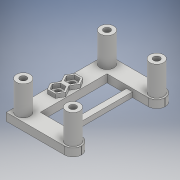
# Autodesk Inventor part: mountMount
Saved by Autodesk Inventor 2018 (Build 220112000, 112)
## iProperties
Created: 2018-05-09
Part Number: mountMount
Material: Generic
Document SubType Name: Modeling
Designer: s4321966
Density: 1 g/cm^3
Appearance: Default
Mass: 5.25986 g
Surface Area: 52.6128 cm^2
Volume: 5.25986 cm^3
Author: s4321966
Autodesk Inventor part; units mm, degrees
ref_plane "YZ Plane" through (0, 0, 0) normal (1, 0, 0) x (0, 1, 0)
ref_plane "XZ Plane" through (0, 0, 0) normal (0, 1, 0) x (-1, 0, 0)
ref_plane "XY Plane" through (0, 0, 0) normal (0, 0, 1) x (1, 0, 0)
sketch "Sketch1" plane through (0, 0, 0) normal (0, 0, 1) x (1, 0, 0)
  line L0 (0, 0) -> (41.5, 0)
  line L1 (41.5, 0) -> (41.5, -73)
  line L2 (41.5, -73) -> (0, -73)
  line L3 (0, -73) -> (0, 0)
  line L4 (0, -73) -> (3.11, -73)
  line L5 (0, -73) -> (3.11, -73) construction
  line L6 (3.11, -73) -> (3.11, -69.85)
  line L7 (3.11, -73) -> (6.26, -73) construction
  line L8 (3.11, -69.85) -> (14.54, -69.85)
  line L9 (14.54, -69.85) -> (19.65, -69.85)
  line L10 (19.65, -69.85) -> (31.08, -69.85)
  circle A0 centre (3.11, -69.85) radius 1.6
  circle A1 centre (14.54, -69.85) radius 1.6
  circle A2 centre (19.65, -69.85) radius 1.6
  circle A3 centre (31.08, -69.85) radius 1.6
  line L11 (3.11, -69.85) -> (3.11, -55.42)
  line L12 (3.11, -69.85) -> (17.54, -69.85) construction
  line L13 (0, -73) -> (4.33, -73)
  line L14 (0, -73) -> (4.33, -73) construction
  line L15 (4.33, -73) -> (4.33, -53.49)
  line L16 (3.11, -55.42) -> (6.6479, -55.42)
  circle A4 centre (4.33, -55.42) radius 1.651
  line L17 (4.33, -55.42) -> (4.33, -37.69)
  line L18 (4.33, -55.42) -> (22.06, -55.42) construction
  line L19 (4.33, -55.42) -> (29.68, -55.42)
  line L20 (4.33, -55.42) -> (29.68, -55.42) construction
  circle A5 centre (4.33, -37.69) radius 1.651
  circle A6 centre (29.68, -55.42) radius 1.651
  line L21 (4.33, -37.69) -> (39.0376, -37.69)
  line L22 (29.68, -55.42) -> (29.68, -25.3245)
  circle A7 centre (29.68, -37.69) radius 1.651
  line L23 (4.33, -37.69) -> (4.33, -30.44)
  line L24 (4.33, -37.69) -> (11.58, -37.69) construction
  line L25 (4.33, -30.44) -> (4.33, -12.71)
  line L26 (4.33, -30.44) -> (29.68, -30.44)
  line L27 (4.33, -30.44) -> (29.68, -30.44) construction
  line L28 (4.33, -12.71) -> (29.68, -12.71)
  circle A8 centre (29.68, -12.71) radius 1.651
  circle A9 centre (4.33, -12.71) radius 1.651
  circle A10 centre (4.33, -30.44) radius 1.651
  circle A11 centre (29.68, -30.44) radius 1.651
  line L29 (29.68, -12.71) -> (29.68, -11.3536)
  dimension "d0" = 41.5
  dimension "d1" = 73
  dimension "d2" = 3.11
  dimension "d3" = 0
  dimension "d4" = 3.15
  dimension "d5" = 90
  dimension "d6" = 11.43
  dimension "d7" = 90
  dimension "d9" = 5.11
  dimension "d10" = 11.43
  dimension "d11" = 180
  dimension "d12" = 3.2
  dimension "d13" = 3.2
  dimension "d14" = 3.2
  dimension "d15" = 3.2
  dimension "d18" = 14.43
  dimension "d19" = 90
  dimension "d20" = 4.33
  dimension "d21" = 0
  dimension "d22" = 3.302
  dimension "d23" = 17.73
  dimension "d24" = 90
  dimension "d25" = 25.35
  dimension "d26" = 0
  dimension "d27" = 3.302
  dimension "d28" = 3.302
  dimension "d29" = 3.302
  dimension "d30" = 7.25
  dimension "d31" = 90
  dimension "d32" = 17.73
  dimension "d33" = 180
  dimension "d34" = 25.35
  dimension "d35" = 0
  dimension "d36" = 25.35
  dimension "d37" = 3.302
  dimension "d38" = 3.302
  dimension "d39" = 3.302
  dimension "d40" = 3.302
  constraints: 60 end point, 15 horizontal, 12 centre point, 9 coincident, 8 equal length, 5 perpendicular, 5 vertical, 4 point on line, 3 collinear, 2 parallel
  measures "d0" distance of L1.end L2.end
  measures "d1" distance of L0.end L1.end
  measures "d2" distance of L2.end L4.end
  measures "d3" distance between parallel lines of L4 L5
  measures "d4" distance of L4.end L6.end
  measures "d5" angle of L7 L6
  measures "d6" distance of L6.end L8.end
  measures "d7" angle of L6 L8
  measures "d9" distance of L8.end L9.end
  measures "d10" distance of L9.end L10.end
  measures "d11" angle of L10 L9
  measures "d12" diameter of A0
  measures "d13" diameter of A1
  measures "d14" diameter of A2
  measures "d15" diameter of A3
  measures "d18" distance of L11.start L11.end
  measures "d19" angle of L12 L11
  measures "d20" distance of L2.end L13.end
  measures "d21" distance between parallel lines of L13 L14
  measures "d22" diameter of A4
  measures "d23" distance of L17.start L17.end
  measures "d24" angle of L18 L17
  measures "d25" distance of L17.start L19.end
  measures "d26" distance between parallel lines of L19 L20
  measures "d27" diameter of A5
  measures "d28" diameter of A6
  measures "d29" diameter of A7
  measures "d30" distance of L21.start L23.end
  measures "d31" angle of L24 L23
  measures "d32" distance of L23.end L25.end
  measures "d33" angle of L25 L23
  measures "d34" distance of L23.end L26.end
  measures "d35" distance between parallel lines of L26 L27
  measures "d36" distance of L25.end L28.end
  measures "d37" diameter of A8
  measures "d38" diameter of A9
  measures "d39" diameter of A10
  measures "d40" diameter of A11
extrude "Extrusion2" add sketch "Sketch1" along normal blind 4 contours L0 L1 L2 L15 A0 A4 L16 L19 A6 L22 A7 A11 L26 A10 L23 A5 L17 L11 L6 L3 | L6 A0 L15 L2 | L11 A4 L15 A0 | L15 L17 A5 L21 A7 L22 A6 L19 L16 A4 | L23 A10 L26 A11 L22 A7 L21 A5
sketch "Sketch3" plane through (0, 0, 4) normal (0, 0, 1) x (1, 0, 0)
  circle A0 centre (4.33, -55.42) radius 1.651 projected
  circle A1 centre (4.33, -55.42) radius 3.5
  circle A2 centre (29.68, -55.42) radius 1.651 projected
  circle A3 centre (29.68, -55.42) radius 3.5
  circle A4 centre (4.33, -12.71) radius 1.651 projected
  circle A5 centre (4.33, -12.71) radius 3.5
  circle A6 centre (29.68, -12.71) radius 1.651 projected
  circle A7 centre (29.68, -12.71) radius 3.5
  point P0 (0, 0)
  dimension "d46" = 7
  dimension "d47" = 7
  dimension "d48" = 7
  dimension "d49" = 7
  constraints: 4 centre point, 4 coincident
  measures "d46" diameter of A1
  measures "d47" diameter of A3
  measures "d48" diameter of A5
  measures "d49" diameter of A7
extrude "Extrusion4" add sketch "Sketch3" along normal blind 15
sketch "Sketch8" plane through (0, 0, 0) normal (0, 0, -1) x (-1, 0, 0)
  circle A0 centre (-4.33, -12.71) radius 1.651 projected
  circle A1 centre (-4.33, -12.71) radius 3
  circle A2 centre (-29.68, -12.71) radius 1.651 projected
  circle A3 centre (-29.68, -12.71) radius 3
  circle A4 centre (-29.68, -55.42) radius 1.651 projected
  circle A5 centre (-29.68, -55.42) radius 3
  circle A6 centre (-4.33, -55.42) radius 1.651 projected
  circle A7 centre (-4.33, -55.42) radius 3
  line L0 (-1.33, -12.71) -> (-2.83, -15.3081)
  line L1 (-2.83, -15.3081) -> (-5.83, -15.3081)
  line L2 (-5.83, -15.3081) -> (-7.33, -12.71)
  line L3 (-7.33, -12.71) -> (-5.83, -10.1119)
  line L4 (-5.83, -10.1119) -> (-2.83, -10.1119)
  line L5 (-2.83, -10.1119) -> (-1.33, -12.71)
  circle A8 centre (-29.68, -12.71) radius 3.5 projected
  line L6 (-26.18, -12.6978) -> (-27.9194, -15.735)
  line L7 (-27.9194, -15.735) -> (-31.4194, -15.7472)
  line L8 (-31.4194, -15.7472) -> (-33.18, -12.7222)
  line L9 (-33.18, -12.7222) -> (-31.4406, -9.685)
  line L10 (-31.4406, -9.685) -> (-27.9406, -9.6728)
  line L11 (-27.9406, -9.6728) -> (-26.18, -12.6978)
  line L12 (-26.68, -55.42) -> (-28.18, -58.0181)
  line L13 (-28.18, -58.0181) -> (-31.18, -58.0181)
  line L14 (-31.18, -58.0181) -> (-32.68, -55.42)
  line L15 (-32.68, -55.42) -> (-31.18, -52.8219)
  line L16 (-31.18, -52.8219) -> (-28.18, -52.8219)
  line L17 (-28.18, -52.8219) -> (-26.68, -55.42)
  line L18 (-1.3301, -55.3946) -> (-2.808, -58.0053)
  line L19 (-2.808, -58.0053) -> (-5.8079, -58.0307)
  line L20 (-5.8079, -58.0307) -> (-7.3299, -55.4454)
  line L21 (-7.3299, -55.4454) -> (-5.852, -52.8347)
  line L22 (-5.852, -52.8347) -> (-2.8521, -52.8093)
  line L23 (-2.8521, -52.8093) -> (-1.3301, -55.3946)
  point P0 (0, 0)
  dimension "d53" = 6
  dimension "d55" = 6
  dimension "d56" = 6
  dimension "d54" = 6
  constraints: 48 end point, 8 coincident, 2 horizontal alignment, 1 centre point, 1 point on line, 61 other
  measures "d54" diameter of A3
extrude "Extrusion5" cut sketch "Sketch8" against normal blind 2 contours L0 L1 L2 L3 L4 L5 | A2 | A3 | L12 L13 L14 L15 L16 L17 | L18 L19 L20 L21 L22 L23 | L6 L7 L8 L9 L10 L11
sketch "Sketch9" plane through (0, 0, 4) normal (0, 0, 1) x (1, 0, 0)
  circle A0 centre (4.33, -30.44) radius 1.651 projected
  circle A1 centre (4.33, -30.44) radius 1.651
  circle A2 centre (4.33, -37.69) radius 1.651 projected
  circle A3 centre (4.33, -37.69) radius 1.651
  line L0 (7.33, -30.44) -> (5.83, -33.0381)
  line L1 (5.83, -33.0381) -> (2.83, -33.0381)
  line L2 (2.83, -33.0381) -> (1.33, -30.44)
  line L3 (1.33, -30.44) -> (2.83, -27.8419)
  line L4 (2.83, -27.8419) -> (5.83, -27.8419)
  line L5 (5.83, -27.8419) -> (7.33, -30.44)
  line L6 (7.33, -37.69) -> (5.83, -40.2881)
  line L7 (5.83, -40.2881) -> (2.83, -40.2881)
  line L8 (2.83, -40.2881) -> (1.33, -37.69)
  line L9 (1.33, -37.69) -> (2.83, -35.0919)
  line L10 (2.83, -35.0919) -> (5.83, -35.0919)
  line L11 (5.83, -35.0919) -> (7.33, -37.69)
  line L12 (8.33, -30.44) -> (6.33, -33.9041)
  line L13 (6.33, -33.9041) -> (2.33, -33.9041)
  line L14 (2.33, -33.9041) -> (0.33, -30.44)
  line L15 (0.33, -30.44) -> (2.33, -26.9759)
  line L16 (2.33, -26.9759) -> (6.33, -26.9759)
  line L17 (6.33, -26.9759) -> (8.33, -30.44)
  line L18 (8.33, -37.69) -> (6.33, -41.1541)
  line L19 (6.33, -41.1541) -> (2.33, -41.1541)
  line L20 (2.33, -41.1541) -> (0.33, -37.69)
  line L21 (0.33, -37.69) -> (2.33, -34.2259)
  line L22 (2.33, -34.2259) -> (6.33, -34.2259)
  line L23 (6.33, -34.2259) -> (8.33, -37.69)
  line L24 (6.33, -33.9041) -> (6.33, -34.2259)
  line L25 (2.33, -33.9041) -> (2.33, -34.2259)
  point P0 (0, 0)
  dimension "d59" = 3.302
  dimension "d60" = 3.302
  constraints: 52 end point, 2 centre point, 2 coincident, 2 vertical, 1 point on line, 52 other
  measures "d59" diameter of A1
  measures "d60" diameter of A3
extrude "Extrusion6" add sketch "Sketch9" along normal blind 2 contours L12 L13 L14 L15 L16 L17 | L24 L22 L25 L13 | L23 L18 L19 L20 L21 L22
sketch "Sketch10" plane through (0, 0, 0) normal (0, 0, -1) x (-1, 0, 0)
  circle A0 centre (-4.33, -55.42) radius 1.651 projected
  circle A1 centre (-4.33, -12.71) radius 3.5 projected
  circle A2 centre (-4.33, -12.71) radius 4.33
  line L0 (-4.33, -8.38) -> (6.0992, -8.38)
  line L1 (-4.33, -8.38) -> (-46.273, -8.38)
  circle A3 centre (-29.68, -55.42) radius 1.651 projected
  circle A4 centre (-29.68, -12.71) radius 1.651 projected
  circle A5 centre (-29.68, -12.71) radius 4.33
  line L2 (-34.01, -12.71) -> (-34.01, 23.2585)
  circle A6 centre (-4.33, -55.42) radius 4.33
  line L3 (-34.01, -12.71) -> (-34.01, -66.3278)
  line L4 (-4.33, -59.75) -> (-38.3543, -59.75)
  circle A7 centre (-29.68, -55.42) radius 4.33
  line L5 (-29.68, -55.42) -> (-29.68, -12.71)
  circle A8 centre (-4.33, -12.71) radius 1.651 projected
  line L6 (-4.33, -12.71) -> (-29.68, -12.71)
  line L7 (-18.2288, -59.75) -> (-46.273, -59.75)
  line L8 (-46.273, -59.75) -> (-46.273, -78.0952)
  line L9 (-46.273, -78.0952) -> (-18.2288, -78.0952)
  line L10 (-18.2288, -78.0952) -> (-18.2288, -59.75)
  line L11 (-18.2288, -59.75) -> (2.2846, -59.75)
  line L12 (2.2846, -59.75) -> (2.2846, -79.2844)
  line L13 (2.2846, -79.2844) -> (-18.2288, -79.2844)
  line L14 (-18.2288, -79.2844) -> (-18.2288, -59.75)
  line L15 (-34.01, -59.75) -> (-49.3705, -59.75)
  line L16 (-49.3705, -59.75) -> (-49.3705, 18.5259)
  line L17 (-49.3705, 18.5259) -> (-34.01, 18.5259)
  line L18 (-34.01, 18.5259) -> (-34.01, -59.75)
  line L19 (-34.01, -8.38) -> (8.0076, -8.38)
  line L20 (8.0076, -8.38) -> (8.0076, 15.8503)
  line L21 (8.0076, 15.8503) -> (-34.01, 15.8503)
  line L22 (-34.01, 15.8503) -> (-34.01, -8.38)
  point P0 (0, 0)
  constraints: 46 end point, 8 horizontal, 8 parallel, 6 point on line, 5 perpendicular, 4 coincident, 4 vertical, 2 vertical alignment, 1 centre point, 1 horizontal alignment, 1 tangent, 6 other
extrude "Extrusion7" cut sketch "Sketch10" along normal mid plane 100 contours L1 L2 L21 L20 L19 L0 | L2 L3 L4 L7 L15 L16 L17 | L4 L10 L9 L8 L7 | L4 L11 L12 L13 L14 L10
sketch "Sketch11" plane through (0, 0, 0) normal (0, 0, -1) x (-1, 0, 0)
  line L0 (-34.01, -59.75) -> (0, -59.75) projected
  line L1 (0, -8.38) -> (-34.01, -8.38) projected
  circle A0 centre (-4.33, -55.42) radius 1.651 projected
  circle A1 centre (-4.33, -55.42) radius 4.3403
  circle A2 centre (-4.33, -12.71) radius 1.651 projected
  circle A3 centre (-4.33, -12.71) radius 4.3403
  line L2 (-4.3352, -51.0797) -> (-29.68, -51.0797)
  line L3 (-29.68, -59.75) -> (-4.3352, -59.75)
  line L4 (-4.3352, -59.75) -> (-4.3352, -51.0797)
  line L5 (-4.3352, -17.0503) -> (-29.68, -17.0503)
  line L6 (-29.68, -8.38) -> (-4.3352, -8.38)
  line L7 (-4.3352, -8.38) -> (-4.3352, -17.0503)
  line L8 (-4.3352, -51.0797) -> (-8.6703, -51.0797)
  line L9 (-8.6703, -51.0797) -> (-8.6703, -12.7152)
  line L10 (-8.6703, -12.7152) -> (-4.3352, -12.7152)
  line L11 (-4.3352, -12.7152) -> (-4.3352, -51.0797)
  line L12 (-34.01, -8.38) -> (-34.01, -59.75) projected
  line L13 (-8.6703, -17.0503) -> (-34.01, -17.0503)
  line L14 (-34.01, -17.0503) -> (-34.01, -51.0797)
  line L15 (-34.01, -51.0797) -> (-8.6703, -51.0797)
  line L16 (-8.6703, -51.0797) -> (-8.6703, -17.0503)
  line L17 (-29.68, -59.75) -> (-36.7019, -59.75)
  line L18 (-36.7019, -59.75) -> (-36.7019, -51.0797)
  line L19 (-36.7019, -51.0797) -> (-29.68, -51.0797)
  line L20 (-29.68, -17.0503) -> (-34.01, -17.0503)
  line L21 (-34.01, -17.0503) -> (-34.01, -8.38)
  line L22 (-34.01, -8.38) -> (-29.68, -8.38)
  arc A4 (-29.68, -51.0797) -> (-29.68, -59.75) centre (-29.68, -55.4148) ccw
  arc A5 (-29.68, -8.38) -> (-29.68, -17.0503) centre (-29.68, -12.7152) ccw
  line L23 (-29.68, -17.0503) -> (-40.5173, -17.0503)
  line L24 (-40.5173, -17.0503) -> (-40.5173, -8.38)
  line L25 (-40.5173, -8.38) -> (-29.68, -8.38)
  line L26 (-8.6703, -51.0797) -> (-41.5169, -51.0797)
  line L27 (-41.5169, -51.0797) -> (-41.5169, -17.0503)
  line L28 (-41.5169, -17.0503) -> (-8.6703, -17.0503)
  line L29 (-8.6703, -17.0503) -> (-8.6703, -51.0797)
  arc A6 (-29.68, -8.38) -> (-29.68, -17.0503) centre (-29.68, -12.7152) ccw
  line L30 (-29.68, -8.38) -> (-34.01, -8.38)
  point P0 (0, 0)
  point P1 (-29.68, -55.42)
  constraints: 56 end point, 11 parallel, 8 horizontal, 8 point on circle, 7 point on line, 6 perpendicular, 4 centre point, 2 coincident, 2 tangent, 1 collinear, 3 other
extrude "Extrusion8" cut sketch "Sketch11" along normal mid plane 100 contours L12 A4 L0 | L17 L18 L19 L12 A4 | L12 L15 A4 | L12 L13 L5 L9 L2 L15 | L23 L24 L25 L12 A5 | L12 A5 L13 | L12 L1 A5
sketch "Sketch12" plane through (0, 0, 0) normal (0, 0, -1) x (-1, 0, 0)
  line L0 (-29.68, -51.0797) -> (-8.6703, -51.0797) projected
  line L1 (-8.6703, -17.0503) -> (-29.68, -17.0503) projected
  line L2 (-8.6703, -51.0797) -> (-18.6703, -51.0797)
  line L3 (-18.6703, -51.0797) -> (-18.6703, -17.0503)
  line L4 (-18.6703, -17.0503) -> (-8.6703, -17.0503)
  line L5 (-8.6703, -17.0503) -> (-8.6703, -51.0797)
  line L6 (-18.6703, -17.0503) -> (-21.6703, -17.0503)
  line L7 (-21.6703, -17.0503) -> (-21.6703, -51.0797)
  line L8 (-21.6703, -51.0797) -> (-18.6703, -51.0797)
  line L9 (-18.6703, -51.0797) -> (-18.6703, -17.0503)
  point P0 (0, 0)
  dimension "d71" = 10
  dimension "d72" = 3
  constraints: 16 end point, 4 parallel, 2 horizontal, 2 perpendicular, 2 point on line
  measures "d71" distance of L3.end L4.end
  measures "d72" distance of L8.end L7.end
extrude "Extrusion9" add sketch "Sketch12" against normal blind 2.5 contours L7 L1 L3 L0
body "Solid2"
